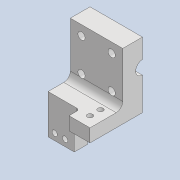
# Autodesk Inventor part: 0008-10-046 Fixare axa si port cablu
Saved by Autodesk Inventor 2020 (Build 240168000, 168)
## iProperties
Created: 2021-02-27
Part Number: 0008-10-046 Fixare axa si port cablu
Material: Generic
Document SubType Name: Modeling
Designer: Iulian Bors
Density: 1 g/cm^3
Appearance: Default
Description: Fixare Axa si portcablu
Mass: 37.7086 g
Surface Area: 110.347 cm^2
Volume: 37.7086 cm^3
Author: Iulian Bors
Subject: 046
Autodesk Inventor part; units mm, degrees
ref_plane "YZ Plane" through (0, 0, 0) normal (1, 0, 0) x (0, 1, 0)
ref_plane "XZ Plane" through (0, 0, 0) normal (0, 1, 0) x (-1, 0, 0)
ref_plane "XY Plane" through (0, 0, 0) normal (0, 0, 1) x (1, 0, 0)
sketch "Sketch1" plane through (0, 0, 0) normal (0, 0, 1) x (1, 0, 0)
  line L0 (-20, 20) -> (20, 20)
  line L1 (20, 20) -> (20, -20)
  line L2 (20, -20) -> (-20, -20)
  line L3 (-20, -20) -> (-20, 20)
  point P0 (0, 0)
  point P1 (-20, 0)
  point P2 (0, 20)
  dimension "d0" = 40
  dimension "d1" = 40
  constraints: 8 end point, 2 midpoint, 2 parallel, 1 horizontal, 1 horizontal alignment, 1 perpendicular, 1 vertical alignment
  measures "d0" distance of L2.end L0.start
  measures "d1" distance of L0.start L0.end
extrude "Extrusion1" add sketch "Sketch1" along normal blind 15
sketch "Sketch2" plane through (-20, -20, 0) normal (-1, 0, 0) x (0, 0, 1)
  circle A0 centre (0, 20) radius 5.15
  line L0 (0, 40) -> (0, 0) projected
  dimension "d5" = 10.3
  dimension "d8" = 0
  constraints: 1 centre point, 1 coincident, 1 midpoint
  measures "d5" diameter of A0
  measures "d8" distance of point (0, 20) A0.centre
extrude "Extrusion2" cut sketch "Sketch2" against normal through all
sketch "Sketch3" plane through (0, 0, 0) normal (0, 0, -1) x (-1, 0, 0)
  line L0 (-20, 5.15) -> (-20, 20) projected
  line L1 (-20, -20) -> (-20, -5.15) projected
  line L2 (20, -20) -> (-20, -20) projected
  line L3 (-20, 20) -> (20, 20) projected
  line L4 (20, -5.15) -> (20, -20) projected
  point P0 (0, 0)
  point P1 (-11.5, -12.575)
  point P2 (-11.5, 12.575)
  point P3 (-20, 12.575)
  point P4 (-20, -12.575)
  point P5 (0, 20)
  point P6 (11.5, -12.575)
  point P7 (11.5, 12.575)
  dimension "d20" = 8.5
  dimension "d21" = 8.5
  constraints: 4 horizontal alignment, 3 midpoint, 2 vertical alignment
  measures "d20" distance from line of L1 point (-11.5, -12.575)
  measures "d21" distance from line of point (11.5, -12.575) L4
hole "Hole1" at (11.5, -12.575, 0) at (11.5, 12.575, 0) at (-11.5, -12.575, 0) at (-11.5, 12.575, 0) direction (0, 0, 1) diameter 5.5 end through all
sketch "Sketch4" plane through (-20, -20, 0) normal (0, -1, 0) x (1, 0, 0)
  line L0 (40, 0) -> (0, 0)
  line L1 (0, 0) -> (0, 40)
  line L2 (0, 40) -> (40, 40)
  line L3 (40, 40) -> (40, 0)
  line L4 (0, 0) -> (40, 0) projected
  line L5 (0, 0) -> (0, 15) projected
  line L6 (40, 0) -> (40, 15) projected
  point P0 (20, 0)
  dimension "d22" = 40
  constraints: 8 end point, 3 collinear, 2 parallel, 1 horizontal, 1 perpendicular
  measures "d22" distance between parallel lines of L2 L0
extrude "Extrusion3" add sketch "Sketch4" along normal blind 10
fillet "Fillet2" radius 5 1 edges at (0, -20, 15)
sketch "Sketch5" plane through (-20, -20, 0) normal (0, 1, 0) x (1, 0, 0)
  line L0 (40, -40) -> (0, -40) projected
  line L1 (40, -20) -> (40, -40) projected
  point P0 (20, 0)
  point P1 (32, -32)
  point P2 (32, -24)
  dimension "d26" = 8
  dimension "d42" = 8
  constraints: 1 vertical alignment
  measures "d26" distance of point (32, -24) point (32, -32)
  measures "d42" distance from line of L1 point (32, -32)
hole "Hole2" at (12, -20, 32) at (12, -20, 24) direction (0, -1, 0) diameter 4 end through all
sketch "Sketch7" plane through (-20, -30, 0) normal (0, -1, 0) x (1, 0, 0)
  line L0 (20, 22) -> (0, 22)
  line L1 (0, 22) -> (0, 32)
  line L2 (0, 32) -> (20, 32)
  line L3 (20, 32) -> (20, 22)
  line L4 (40, 40) -> (0, 40) projected
  line L5 (0, 40) -> (0, 0) projected
  point P0 (20, 0)
  dimension "d37" = 8
  dimension "d38" = 20
  dimension "d39" = 10
  constraints: 8 end point, 2 parallel, 1 collinear, 1 horizontal, 1 perpendicular
  measures "d37" distance between parallel lines of L2 L4
  measures "d38" distance of L0.start L0.end
  measures "d39" distance of L0.end L1.end
extrude "Extrusion4" add sketch "Sketch7" along normal blind 20
sketch "Sketch8" plane through (-20, -30, 32) normal (0, 0, 1) x (1, 0, 0)
  line L0 (0, 0) -> (0, -20) projected
  line L1 (20, -20) -> (0, -20) projected
  point P0 (20, 30)
  point P1 (5, -15)
  point P2 (13, -15)
  point P3 (0, -10)
  dimension "d43" = 5
  dimension "d44" = 8
  dimension "d56" = 5
  constraints: 1 horizontal alignment, 1 midpoint
  measures "d43" distance from line of L0 point (5, -15)
  measures "d44" distance of point (5, -15) point (13, -15)
  measures "d56" distance from line of point (5, -15) L1
hole "Hole3" at (-15, -45, 32) at (-7, -45, 32) direction (0, 0, -1) diameter 4 end through all
sketch "Sketch9" plane through (-20, -30, 0) normal (0, -1, 0) x (1, 0, 0)
  line L0 (24, 32) -> (0, 32)
  line L1 (0, 32) -> (0, 40)
  line L2 (0, 40) -> (24, 40)
  line L3 (24, 40) -> (24, 32)
  circle A0 centre (32, 32) radius 2 projected
  line L4 (20, 32) -> (0, 32) projected
  line L5 (40, 40) -> (0, 40) projected
  line L6 (0, 40) -> (0, 32) projected
  point P0 (20, 0)
  dimension "d52" = 8
  constraints: 8 end point, 3 collinear, 2 parallel, 1 horizontal, 1 perpendicular
  measures "d52" distance from line of A0.centre L3
extrude "Extrusion5" cut sketch "Sketch9" against normal through all contours L0 L1 L2 L3
fillet "Fillet3" radius 2 1 edges at (4, -25, 32)
equation "\"d21\" = d20"
body "Solid1"
